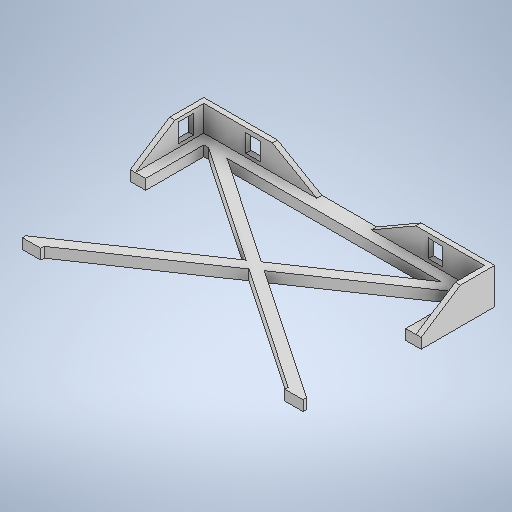
# Autodesk Inventor part: Part6
Saved by Autodesk Inventor 2025.2 (Build 292293000, 293)
## iProperties
Created: 2025-01-22
Part Number: Part6
Material: Generic
Document SubType Name: Modeling
Designer: 24oscnor
Density: 1 g/cm^3
Appearance: Default
Author: 24oscnor
Autodesk Inventor part; units mm, degrees
ref_plane "YZ Plane" through (0, 0, 0) normal (1, 0, 0) x (0, 1, 0)
ref_plane "XZ Plane" through (0, 0, 0) normal (0, 1, 0) x (-1, 0, 0)
ref_plane "XY Plane" through (0, 0, 0) normal (0, 0, 1) x (1, 0, 0)
sketch "Sketch1" plane through (0, 0, 0) normal (0, 1, 0) x (-1, 0, 0)
  line L0 (82, 0) -> (82, -52)
  line L1 (82, -52) -> (0, -52)
  line L2 (0, -52) -> (0, 0)
  line L3 (82, 0) -> (0, 0)
  line L4 (0, 0) -> (76.656, -52)
  line L5 (82, -52) -> (5.344, 0)
  line L6 (82, -26) -> (0, -26) construction
  line L7 (0, -52) -> (76.656, 0)
  line L8 (82, 0) -> (5.344, -52)
  line L9 (41, -52) -> (41, 0) construction
  line L10 (82, -49) -> (0, -49)
  line L11 (3, -52) -> (3, -32)
  line L12 (3, -32) -> (0, -32)
  line L13 (79, -52) -> (79, -32)
  line L14 (79, -32) -> (82, -32)
  line L15 (76.656, 0) -> (76.656, 1)
  line L16 (76.656, 1) -> (82, 1)
  line L17 (82, 1) -> (82, 0)
  line L18 (5.344, 0) -> (5.344, 1)
  line L19 (5.344, 1) -> (0, 1)
  line L20 (0, 1) -> (0, 0)
  point P0 (43.672, -26)
  point P1 (41, -24.1874)
  point P2 (38.328, -26)
  point P3 (4.4225, -49)
  point P4 (0, -49)
  point P5 (77.5775, -49)
  point P6 (41, -27.8126)
  point P7 (72.2336, -49)
  point P8 (9.7664, -49)
  point P9 (79, -49)
  point P10 (3, -49)
  dimension "d5" = 82
  dimension "d6" = 52
  dimension "d7" = 3
  dimension "d9" = 3
  dimension "d12" = 20
  dimension "d13" = 3
  dimension "d14" = 20
  dimension "d15" = 3
  dimension "d35" = 1
  constraints: 42 end point, 6 point on line, 5 perpendicular, 4 midpoint, 4 parallel, 4 symmetric about line, 3 vertical, 1 horizontal
  measures "d5" distance between parallel lines of L0 L2
  measures "d6" distance from line of L2.end L1
  measures "d7" distance between parallel lines of L5 L4
  measures "d9" distance between parallel lines of L10 L1
  measures "d12" distance of L11.start L11.end
  measures "d13" distance of L11.end L12.end
  measures "d14" distance of L13.start L13.end
  measures "d15" distance between parallel lines of L0 L13
  measures "d35" distance of L7.end L15.end
extrude "Extrusion1" add sketch "Sketch1" along normal blind 3 contours L8 L5 L7 L3 | L3 L15 L16 L17 | L0 L10 L13 L14 | L8 L4 L7 L5 | L5 L10 L4 L8 | L0 L5 L13 L10 | L5 L7 L4 L3 | L3 L20 L19 L18 | L10 L13 L5 | L5 L13 L1 L4 L10 | L8 L10 L7 L4 | L1 L13 L5 | L4 L1 L8 L10 | L8 L1 L11 L7 L10 | L12 L11 L10 L2 | L7 L11 L10 | L10 L11 L7 L2 | L11 L1 L7
sketch "Sketch2" plane through (0, 0, -52) normal (0, 0, -1) x (-1, 0, 0)
  line L0 (0, 3) -> (38.328, 3) projected
  line L1 (82, 0) -> (76.656, 0) projected
  line L2 (0, 3) -> (82, 3)
  line L3 (82, 3) -> (82, 0)
  line L4 (82, 0) -> (0, 0)
  line L5 (0, 0) -> (0, 3)
  line L6 (0, 3) -> (0, 10.5)
  line L7 (0, 10.5) -> (20, 10.5)
  line L8 (20, 10.5) -> (32.9904, 3)
  line L9 (12.24, 9.2) -> (16.44, 9.2)
  line L10 (16.44, 9.2) -> (16.44, 4)
  line L11 (16.44, 4) -> (12.24, 4)
  line L12 (12.24, 4) -> (12.24, 9.2)
  line L13 (41, 0) -> (41, 19.2831) construction
  line L14 (32.9904, 3) -> (41, 3) construction
  line L15 (82, 3) -> (43.672, 3)
  line L16 (82, 3) -> (0, 3)
  line L17 (82, 0) -> (82, 3)
  line L18 (82, 3) -> (82, 10.5)
  line L19 (82, 10.5) -> (62, 10.5)
  line L20 (62, 10.5) -> (49.0096, 3)
  line L21 (69.76, 9.2) -> (65.56, 9.2)
  line L22 (65.56, 9.2) -> (65.56, 4)
  line L23 (65.56, 4) -> (69.76, 4)
  line L24 (69.76, 4) -> (69.76, 9.2)
  line L25 (49.0096, 3) -> (41, 3) construction
  point P0 (12.24, 6.6)
  point P1 (14.34, 4)
  point P2 (14.34, 9.2)
  point P3 (69.76, 6.6)
  point P4 (67.66, 4)
  point P5 (67.66, 9.2)
  point P6 (38.328, 3)
  dimension "d16" = 20
  dimension "d17" = 7.5
  dimension "d18" = 15
  dimension "d19" = 12.24
  dimension "d20" = 4.2
  dimension "d21" = 5.2
  dimension "d22" = 4
  constraints: 48 end point, 13 symmetric about line, 6 midpoint, 4 parallel, 3 perpendicular, 3 point on line, 2 horizontal, 2 vertical
  measures "d16" distance of L6.end L7.end
  measures "d17" distance of L0.start L6.end
  measures "d18" distance of L7.end L8.end
  measures "d19" distance from line of point (12.24, 6.6) L6
  measures "d20" distance between parallel lines of L12 L10
  measures "d21" distance of point (14.34, 4) point (14.34, 9.2)
  measures "d22" distance between parallel lines of L4 L11
extrude "Extrusion2" add sketch "Sketch2" along normal blind 1.5
sketch "Sketch3" plane through (0, 0, -32) normal (1, 0, 0) x (0, 0, -1)
  line L0 (21.5, 0) -> (21.5, 10.5) projected
  line L1 (21.5, 10.5) -> (11.5, 10.5)
  line L2 (0, 0) -> (21.5, 0) projected
  line L3 (0, 0) -> (0, 3) projected
  line L4 (21.5, 0) -> (0, 0)
  line L5 (0, 0) -> (0, 3)
  line L6 (0, 3) -> (21.5, 3)
  line L7 (21.5, 3) -> (21.5, 0)
  line L8 (11.5, 10.5) -> (0, 3)
  point P0 (-32, 0)
  dimension "d25" = 10
  constraints: 12 end point, 2 horizontal, 2 parallel, 1 perpendicular
  measures "d25" distance of L0.end L1.end
extrude "Extrusion3" add sketch "Sketch3" along normal blind 1.5
sketch "Sketch4" plane through (-82, 0, -32) normal (-1, 0, 0) x (0, 0, 1)
  line L0 (-11.5, 10.5) -> (0, 3) projected
  line L1 (0, 3) -> (-11.5, 10.5)
  line L2 (-20, 10.5) -> (-21.5, 10.5) projected
  line L3 (-11.5, 10.5) -> (-21.5, 10.5)
  line L4 (-21.5, 10.5) -> (-21.5, 0)
  line L5 (-21.5, 0) -> (0, 0)
  line L6 (0, 0) -> (0, 3)
  line L7 (-17, 9.5) -> (-12.5, 9.5)
  line L8 (-12.5, 9.5) -> (-12.5, 4)
  line L9 (-12.5, 4) -> (-17, 4)
  line L10 (-17, 4) -> (-17, 9.5)
  point P0 (32, 0)
  point P1 (-21.5, 5.25)
  point P2 (-20, 10.5)
  dimension "d28" = 4.5
  dimension "d29" = 4.5
  dimension "d30" = 4
  dimension "d31" = 5.5
  dimension "d32" = 1
  constraints: 18 end point, 4 perpendicular, 2 collinear, 2 parallel, 1 horizontal, 1 midpoint
  measures "d28" distance from line of point (-21.5, 5.25) L10
  measures "d29" distance between parallel lines of L8 L10
  measures "d30" distance between parallel lines of L9 L5
  measures "d31" distance between parallel lines of L7 L9
  measures "d32" distance between parallel lines of L3 L7
extrude "Extrusion4" add sketch "Sketch4" along normal blind 1.5
body "Solid1"
